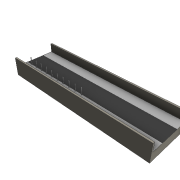
# Autodesk Inventor part: scene2
Saved by Autodesk Inventor 2021 (Build 250183000, 183)
## iProperties
Created: 2022-03-08
Part Number: scene2
Material: Generic
Document SubType Name: Modeling
Designer: Derm
Density: 1 g/cm^3
Appearance: Terrazzo - White-Black
Author: Derm
Autodesk Inventor part; units mm, degrees
ref_plane "YZ Plane" through (0, 0, 0) normal (1, 0, 0) x (0, 1, 0)
ref_plane "XZ Plane" through (0, 0, 0) normal (0, 1, 0) x (-1, 0, 0)
ref_plane "XY Plane" through (0, 0, 0) normal (0, 0, 1) x (1, 0, 0)
sketch "Sketch1" plane through (0, 0, 0) normal (0, 1, 0) x (-1, 0, 0)
  line L0 (50000, 50000) -> (-50000, 50000)
  line L1 (-50000, 50000) -> (-50000, -50000)
  line L2 (-50000, -50000) -> (50000, -50000)
  line L3 (50000, -50000) -> (50000, 50000)
  line L4 (50000, 50000) -> (-50000, -50000) construction
  line L5 (-50000, 50000) -> (50000, -50000) construction
  point P0 (0, 0)
  dimension "d0" = 100000
  dimension "d1" = 100000
  constraints: 12 end point, 2 midpoint, 2 parallel, 1 horizontal, 1 perpendicular
  measures "d0" distance of L1.end L2.end
  measures "d1" distance of L0.end L1.end
extrude "Extrusion1" add sketch "Sketch1" against normal blind 6000
sketch "Sketch2" plane through (0, 0, 0) normal (0, 1, 0) x (1, 0, 0)
  line L0 (50000, -50000) -> (50000, 50000) projected
  line L1 (50000, 50000) -> (-50000, 50000) projected
  line L2 (-50000, 50000) -> (-50000, -50000) projected
  line L3 (-50000, -50000) -> (50000, -50000) projected
  line L4 (50000, 50000) -> (50000, -50000) projected
  line L5 (-50000, -6000) -> (50000, -6000)
  line L6 (50000, -6000) -> (50000, 6000)
  line L7 (-50000, 6000) -> (-50000, -6000)
  line L8 (-50000, -6000) -> (50000, 6000) construction
  line L9 (50000, -6000) -> (-50000, 6000) construction
  line L10 (-50000, 50000) -> (50000, 50000) projected
  line L11 (38735.1966, 9000) -> (38735.1966, 50000)
  line L12 (38735.1966, 50000) -> (27735.1966, 50000)
  line L13 (27735.1966, 50000) -> (27735.1966, 9000)
  line L14 (50000, 6000) -> (41735.1966, 6000)
  line L15 (24735.1966, 6000) -> (-50000, 6000)
  arc A0 (24735.1966, 6000) -> (27735.1966, 9000) centre (24735.1966, 9000) ccw
  arc A1 (38735.1966, 9000) -> (41735.1966, 6000) centre (41735.1966, 9000) ccw
  point P0 (0, 0)
  dimension "d5" = 11000
  dimension "d6" = 3000
  constraints: 20 end point, 4 parallel, 4 point on circle, 4 tangent, 2 centre point, 2 midpoint, 2 point on line, 1 equal radius, 1 horizontal, 1 perpendicular
  measures "d5" distance between parallel lines of L11 L13
  measures "d6" radius of A0
extrude "Extrusion2" cut sketch "Sketch2" against normal blind 100 contours L5 L2 L15 A0 L13 L1 L11 A1 L14 L0
sketch "Sketch3" plane through (0, 0, 0) normal (0, 1, 0) x (1, 0, 0)
  line L0 (50000, 50000) -> (50000, -50000) projected
  line L1 (50000, -50000) -> (-50000, -50000) projected
  line L2 (-50000, -50000) -> (-50000, 50000) projected
  line L3 (-50000, 50000) -> (50000, 50000) projected
  line L4 (-50000, 6000) -> (24735.1966, 6000) projected
  arc A0 (24735.1966, 6000) -> (27735.1966, 9000) centre (24735.1966, 9000) ccw projected
  line L5 (27735.1966, 9000) -> (27735.1966, 50000) projected
  line L6 (27735.1966, 50000) -> (-50000, 50000) projected
  line L7 (-50000, 50000) -> (-50000, 6000) projected
  line L8 (23068.1077, 10876.2035) -> (6908.7226, 10876.2035)
  line L9 (6908.7226, 10876.2035) -> (6908.7226, 28000)
  line L10 (6908.7226, 28000) -> (23068.1077, 28000)
  line L11 (23068.1077, 28000) -> (23068.1077, 10876.2035)
  line L12 (23068.1077, 10876.2035) -> (6908.7226, 28000) construction
  line L13 (6908.7226, 10876.2035) -> (23068.1077, 28000) construction
  point P0 (0, 0)
  point P1 (14988.4151, 19438.1018)
  constraints: 12 end point, 2 midpoint, 2 parallel, 1 horizontal, 1 perpendicular
extrude "Extrusion3" add sketch "Sketch3" along normal blind 5000 contours L8 L9 L10 L11
sketch "Sketch4" plane through (23068.1077, 0, -28000) normal (0, 0, -1) x (-1, 0, 0)
  line L0 (16159.3851, 0) -> (0, 0) projected
  line L1 (16159.3851, 0) -> (16159.3851, 5000) projected
  line L2 (0, 5000) -> (16159.3851, 5000) projected
  line L3 (0, 0) -> (0, 5000) projected
  line L4 (0, 5000) -> (16159.3851, 5000) projected
  line L5 (0, 5000) -> (-502.206, 5000)
  line L6 (-502.206, 5000) -> (1674.3292, 8799.2208)
  line L7 (1674.3292, 8799.2208) -> (8079.6925, 8799.2208)
  line L8 (8079.6925, 5000) -> (8079.6925, 8799.2208)
  line L9 (16159.3851, 5000) -> (16661.5911, 5000)
  line L10 (16661.5911, 5000) -> (14485.0559, 8799.2208)
  line L11 (14485.0559, 8799.2208) -> (8079.6925, 8799.2208)
  point P0 (23068.1077, 0)
  constraints: 14 end point, 2 symmetric about line, 1 horizontal, 1 midpoint, 1 parallel, 1 perpendicular
extrude "Extrusion4" add sketch "Sketch4" against normal up to surface (17123.7965 mm away) contours L2 L8 L11 L10 L9 | L5 L6 L7 L8 L2
sketch "Sketch5" plane through (6908.7226, 0, -10876.2035) normal (0, 0, 1) x (1, 0, 0)
  line L0 (16159.3851, 0) -> (0, 0) projected
  line L1 (16159.3851, 0) -> (16159.3851, 5000) projected
  line L2 (16661.5911, 5000) -> (16159.3851, 5000) projected
  line L3 (14485.0559, 8799.2208) -> (16661.5911, 5000) projected
  line L4 (1674.3292, 8799.2208) -> (14485.0559, 8799.2208) projected
  line L5 (-502.206, 5000) -> (1674.3292, 8799.2208) projected
  line L6 (0, 5000) -> (-502.206, 5000) projected
  line L7 (0, 0) -> (0, 5000) projected
  line L8 (0, 5000) -> (-502.206, 5000) projected
  line L9 (16661.5911, 5000) -> (16159.3851, 5000) projected
  line L10 (0, 5000) -> (16159.3851, 5000)
  point P0 (-6908.7226, 0)
  constraints: 2 end point, 1 collinear
extrude "Extrusion5" add sketch "Sketch5" along normal blind 600 contours L10 L6 L5 L4 L3 L2
ref_plane "Work Plane1" through (23068.1077, 0, -19438.1018) normal (0, 0, -1) x (-1, 0, 0)
mirror "Mirror1" about plane through (23068.1077, 0, -19438.1018) normal (0, 0, -1) of "Extrusion5"
chamfer "Chamfer1" distance 50 angle 45 7 edges at (-12632.4017, 0, -6000) (26856.517, 0, -6878.6797) (27735.1966, 0, -29500) (0, 0, 6000) (38735.1966, 0, -29500) (39613.8763, 0, -6878.6797) (45867.5983, 0, -6000)
chamfer "Chamfer2" distance 3500 angle 45 2 edges at (14988.4151, 8799.2208, -10276.2035) (14988.4151, 8799.2208, -28600)
sketch "Sketch6" plane through (0, 0, 0) normal (0, 1, 0) x (1, 0, 0)
  line L0 (-50000, -6050) -> (50000, -6050) projected
  line L1 (-50000, -6050) -> (-50000, -50000) projected
  line L2 (-50000, -50000) -> (50000, -50000) projected
  line L3 (50000, -50000) -> (50000, -6050) projected
  circle A0 centre (0, -6381.6729) radius 250
  point P0 (0, 0)
  dimension "d21" = 500
  constraints: 1 centre point
  measures "d21" diameter of A0
extrude "Extrusion6" add sketch "Sketch6" along normal blind 5000 contours A0
pattern_linear "Rectangular Pattern1" count 10 spacing 5000 along (-1, 0, 0) of "Extrusion6"
sketch "Sketch7" plane through (0, 0, 0) normal (0, 1, 0) x (1, 0, 0)
  circle A0 centre (-25000, -6381.6729) radius 250 projected
  circle A1 centre (-15000, -6381.6729) radius 250 projected
  circle A2 centre (-5000, -6381.6729) radius 250 projected
  circle A3 centre (-10000, -6381.6729) radius 250 projected
  circle A4 centre (-20000, -6381.6729) radius 250 projected
  circle A5 centre (0, -6381.6729) radius 250 projected
  line L0 (-50000, -6050) -> (50000, -6050) projected
  line L1 (-50000, -6050) -> (-50000, -50000) projected
  line L2 (-50000, -50000) -> (50000, -50000) projected
  line L3 (50000, -50000) -> (50000, -6050) projected
  line L4 (-50000, -6050) -> (-50000, -50000) projected
  line L5 (50000, 50000) -> (50000, -50000) projected
  line L6 (-50000, -14242.1786) -> (50000, -14242.1786)
  line L7 (50000, -14242.1786) -> (50000, -13182.5289)
  line L8 (50000, -13182.5289) -> (-50000, -13182.5289)
  line L9 (-50000, -13182.5289) -> (-50000, -14242.1786)
  circle A6 centre (-30000, -6381.6729) radius 250 projected
  point P0 (0, 0)
  point P1 (-50000, -13182.5289)
  point P2 (50000, -14242.1786)
  constraints: 8 end point, 2 parallel, 2 point on line, 1 horizontal, 1 perpendicular
extrude "Extrusion7" add sketch "Sketch7" along normal blind 6000 contours L8 L3 L6 L1
sketch "Sketch8" plane through (0, 0, 0) normal (0, 0, 1) x (1, 0, 0)
  line L0 (-60036.3598, 14647.1686) -> (68892.7873, 14647.1686)
  line L1 (68892.7873, 14647.1686) -> (68892.7873, -8515.7957)
  line L2 (68892.7873, -8515.7957) -> (-60036.3598, -8515.7957)
  line L3 (-60036.3598, -8515.7957) -> (-60036.3598, 14647.1686)
  point P0 (0, 0)
  constraints: 8 end point, 2 parallel, 1 horizontal, 1 perpendicular
extrude "Extrusion8" cut sketch "Sketch8" against normal through all
mirror "Mirror2" about plane through (4428.2138, 3065.6864, 0) normal (0, 0, -1) of "Extrusion2", "Extrusion1", "Extrusion7"
sketch "Sketch9" plane through (-50000, -100, -6000) normal (0, 1, 0) x (1, 0, 0)
  line L0 (0, -12000) -> (74735.1966, -12000) projected
  arc A0 (77735.1966, -15000) -> (74735.1966, -12000) centre (74735.1966, -15000) ccw projected
  line L1 (77735.1966, -15000) -> (77735.1966, -56000) projected
  line L2 (88735.1966, -56000) -> (77735.1966, -56000) projected
  line L3 (88735.1966, -56000) -> (88735.1966, -15000) projected
  arc A1 (91735.1966, -12000) -> (88735.1966, -15000) centre (91735.1966, -15000) ccw projected
  line L4 (91735.1966, -12000) -> (100000, -12000) projected
  line L5 (100000, 0) -> (100000, -12000) projected
  line L6 (100000, 0) -> (0, 0) projected
  line L7 (0, -12000) -> (0, 0) projected
  arc A2 (77735.1966, -15000) -> (74735.1966, -12000) centre (74735.1966, -15000) ccw projected
  arc A3 (91735.1966, -12000) -> (88735.1966, -15000) centre (91735.1966, -15000) ccw projected
  line L8 (91735.1966, -12000) -> (74735.1966, -12000)
  point P0 (50000, -6000)
  constraints: 2 end point, 2 tangent, 1 horizontal
extrude "Extrusion9" add sketch "Sketch9" along normal up to surface (100 mm away) contours L8 A1 L3 L2 L1 A0
sketch "Sketch10" plane through (-50000, -100, 6000) normal (0, 1, 0) x (1, 0, 0)
  line L0 (0, 0) -> (100000, 0) projected
  line L1 (100000, 12000) -> (100000, 0) projected
  line L2 (100000, 12000) -> (0, 12000) projected
  line L3 (0, 0) -> (0, 12000) projected
  point P0 (50000, 6000)
extrude "Extrusion10" [suppressed]
sketch "Sketch11" plane through (0, 6000, 0) normal (0, 1, 0) x (1, 0, 0)
  line L0 (-50000, -13182.5289) -> (-50000, -14242.1786) projected
  line L1 (-50000, -14242.1786) -> (50000, -14242.1786) projected
  line L2 (50000, -14242.1786) -> (50000, -13182.5289) projected
  line L3 (50000, -13182.5289) -> (-50000, -13182.5289) projected
  line L4 (50000, -13182.5289) -> (-50000, -13182.5289) projected
  line L5 (-50000, -14242.1786) -> (50000, -14242.1786) projected
  line L6 (44357.964, -13182.5289) -> (23293.9294, -13182.5289)
  line L7 (23293.9294, -13182.5289) -> (23293.9294, -14242.1786)
  line L8 (23293.9294, -14242.1786) -> (44357.964, -14242.1786)
  line L9 (44357.964, -14242.1786) -> (44357.964, -13182.5289)
  point P0 (0, 0)
  point P1 (44357.964, -14242.1786)
  constraints: 8 end point, 2 parallel, 2 point on line, 1 horizontal, 1 perpendicular
extrude "Extrusion11" cut sketch "Sketch11" against normal up to surface (6000 mm away) contours L3 L9 L1 L7
sketch "Sketch12" plane through (0, 0, 0) normal (0, 1, 0) x (1, 0, 0)
  line L0 (50000, -6000) -> (-50000, -6000) projected
  line L1 (-50000, -6000) -> (-50000, -13182.5289) projected
  line L2 (-50000, -13182.5289) -> (23293.9294, -13182.5289) projected
  line L3 (23293.9294, -14242.1786) -> (23293.9294, -13182.5289) projected
  line L4 (23293.9294, -14242.1786) -> (-50000, -14242.1786) projected
  line L5 (-50000, -14242.1786) -> (-50000, -50000) projected
  line L6 (-50000, -50000) -> (50000, -50000) projected
  circle A0 centre (-30000, -6381.6729) radius 250 projected
  circle A1 centre (-25000, -6381.6729) radius 250 projected
  circle A2 centre (-20000, -6381.6729) radius 250 projected
  circle A3 centre (-15000, -6381.6729) radius 250 projected
  circle A4 centre (-10000, -6381.6729) radius 250 projected
  circle A5 centre (-5000, -6381.6729) radius 250 projected
  circle A6 centre (0, -6381.6729) radius 250 projected
  line L7 (-50000, 14242.1786) -> (50000, 14242.1786) projected
  line L8 (50000, 14242.1786) -> (50000, 50000) projected
  line L9 (-50000, 50000) -> (50000, 50000) projected
  line L10 (-50000, 50000) -> (-50000, 14242.1786) projected
  line L11 (50000, 13182.5289) -> (-50000, 13182.5289) projected
  line L12 (-50000, 13182.5289) -> (-50000, 6000) projected
  line L13 (-50000, 6000) -> (50000, 6000) projected
  line L14 (50000, 6000) -> (50000, 13182.5289) projected
  line L15 (50000, -6000) -> (-50000, -6000) projected
  line L16 (-50000, -50000) -> (50000, -50000) projected
  line L17 (50000, -50000) -> (50000, -14242.1786) projected
  line L18 (50000, -14242.1786) -> (44357.964, -14242.1786) projected
  line L19 (44357.964, -13182.5289) -> (44357.964, -14242.1786) projected
  line L20 (44357.964, -13182.5289) -> (50000, -13182.5289) projected
  line L21 (50000, -13182.5289) -> (50000, -6000) projected
  line L22 (-50000, -6000) -> (-50000, -13182.5289) projected
  line L23 (-50000, -13182.5289) -> (23293.9294, -13182.5289) projected
  line L24 (23293.9294, -14242.1786) -> (23293.9294, -13182.5289) projected
  line L25 (23293.9294, -14242.1786) -> (-50000, -14242.1786) projected
  line L26 (-50000, -14242.1786) -> (-50000, -50000) projected
  line L27 (50000, -50000) -> (50000, -14242.1786) projected
  line L28 (50000, -14242.1786) -> (44357.964, -14242.1786) projected
  line L29 (44357.964, -13182.5289) -> (44357.964, -14242.1786) projected
  line L30 (44357.964, -13182.5289) -> (50000, -13182.5289) projected
  line L31 (50000, -13182.5289) -> (50000, -6000) projected
  point P0 (0, 0)
extrude "Extrusion12" add sketch "Sketch12" along normal blind 100
sketch "Sketch13" plane through (-50000, -100, -6000) normal (0, 1, 0) x (1, 0, 0)
  line L0 (100000, 0) -> (100000, -12000) projected
  line L1 (100000, 0) -> (0, 0) projected
  line L2 (0, -12000) -> (0, 0) projected
  line L3 (0, -12000) -> (100000, -12000) projected
  point P0 (50000, -6000)
extrude "Extrusion13" add sketch "Sketch13" along normal blind 100
sketch "Sketch15" plane through (23293.9294, 6000, 14242.1786) normal (1, 0, 0) x (0, 0, -1)
  line L0 (0, -5900) -> (1059.6498, -5900) projected
  line L1 (1059.6498, 0) -> (1059.6498, -5900) projected
  line L2 (0, 0) -> (1059.6498, 0) projected
  line L3 (0, -5900) -> (0, 0) projected
  point P0 (14242.1786, -6000)
extrude "Extrusion15" add sketch "Sketch15" along normal up to next
sketch "Sketch16" plane through (0, 100, 0) normal (0, 1, 0) x (1, 0, 0)
  line L0 (-50000, -14242.1786) -> (50000, -14242.1786) projected
  line L1 (-50000, -14242.1786) -> (-50000, -50000) projected
  line L2 (-50000, -50000) -> (50000, -50000) projected
  line L3 (50000, -50000) -> (50000, -14242.1786) projected
  line L4 (50000, 14242.1786) -> (-50000, 14242.1786) projected
  line L5 (50000, 14242.1786) -> (50000, 50000) projected
  line L6 (50000, 50000) -> (-50000, 50000) projected
  line L7 (-50000, 50000) -> (-50000, 14242.1786) projected
  point P0 (0, 0)
extrude "Extrusion16" cut sketch "Sketch16" against normal through all
sketch "Sketch17" plane through (0, 100, 0) normal (0, 1, 0) x (1, 0, 0)
  circle A0 centre (0, -6381.6729) radius 250 projected
  line L0 (-250, -6131.6729) -> (250, -6131.6729)
  line L1 (250, -6131.6729) -> (250, -6631.6729)
  line L2 (250, -6631.6729) -> (-250, -6631.6729)
  line L3 (-250, -6631.6729) -> (-250, -6131.6729)
  circle A1 centre (0, -6381.6729) radius 250 projected
  line L4 (-250, -6131.6729) -> (250, -6631.6729) construction
  line L5 (250, -6131.6729) -> (-250, -6631.6729) construction
  point P0 (0, 0)
  constraints: 12 end point, 2 midpoint, 2 parallel, 1 horizontal, 1 perpendicular
extrude "Extrusion17" [suppressed]
pattern_linear "Rectangular Pattern2" [suppressed]
sketch "Sketch18" plane through (-50000, 0, -6000) normal (0, 1, 0) x (1, 0, 0)
  line L0 (0, 0) -> (0, -12000) projected
  line L1 (100000, -12000) -> (0, -12000) projected
  line L2 (100000, -12000) -> (100000, 0) projected
  line L3 (0, 0) -> (100000, 0) projected
  line L4 (0, -20242.1786) -> (0, 8242.1786) projected
  line L5 (0, -6000) -> (-4058.2639, -6000) construction
  line L6 (0, -6050.8) -> (100000, -6050.8)
  line L7 (100000, -12000) -> (100000, 0) projected
  line L8 (0, -6152.4) -> (100000, -6152.4)
  point P0 (50000, -6000)
  point P1 (0, -6152.4)
  point P2 (100000, -6152.4)
  point P3 (100000, -6050.8)
  dimension "d54" = 50.8
  dimension "d55" = 101.6
  constraints: 6 end point, 4 point on line, 2 perpendicular, 1 horizontal, 1 midpoint
  measures "d54" distance between parallel lines of L6 L5
  measures "d55" distance between parallel lines of L8 L6
extrude "Extrusion18" add sketch "Sketch18" along normal blind 0.254 contours L6 L2 L8 L0
mirror "Mirror3" about plane through (0, 0, 0) normal (0, 0, 1) of "Extrusion18"
sketch "Sketch19" plane through (-50000, 0, -6000) normal (0, 1, 0) x (1, 0, 0)
  line L0 (0, -5847.6) -> (100000, -5847.6) projected
  line L1 (100000, -5847.6) -> (100000, 0) projected
  line L2 (0, 0) -> (100000, 0) projected
  line L3 (0, 0) -> (0, -5847.6) projected
  line L4 (99864.8269, -2873) -> (98950.4269, -2873)
  line L5 (98950.4269, -2873) -> (98950.4269, -2974.6)
  line L6 (98950.4269, -2974.6) -> (99864.8269, -2974.6)
  line L7 (99864.8269, -2974.6) -> (99864.8269, -2873)
  line L8 (99864.8269, -2873) -> (98950.4269, -2974.6) construction
  line L9 (98950.4269, -2873) -> (99864.8269, -2974.6) construction
  point P0 (50000, -6000)
  point P1 (99407.6269, -2923.8)
  dimension "d58" = 101.6
  dimension "d59" = 914.4
  constraints: 12 end point, 2 midpoint, 2 parallel, 1 horizontal, 1 perpendicular
  measures "d58" distance of L6.end L4.start
  measures "d59" distance of L5.end L6.end
extrude "Extrusion19" add sketch "Sketch19" along normal blind 0.254 contours L7 L6 L5 L4
pattern_linear "Rectangular Pattern3" count 31 spacing 3200.4 along (-1, 0, 0) of "Extrusion19"
mirror "Mirror4" about plane through (0, 0, 0) normal (0, 0, 1) of "Extrusion19", "Rectangular Pattern3"
body "Solid1"
